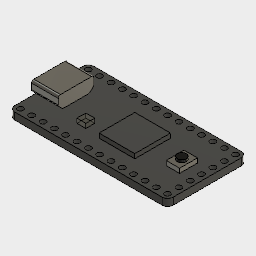
3727 ItsyBitsy M0 (Autodesk Fusion 360 design; units mm, degrees)
Autodesk Fusion 360 part; units mm, degrees
sketch "PCB" plane through (0, 0, 0) normal (0, 0, 1) x (1, 0, 0)
  line L0 (0.508, 6.858) -> (0, 6.35)
  line L1 (0, 16.51) -> (0, 11.684)
  line L2 (0.508, 11.176) -> (0.508, 6.858)
  arc A0 (0, 1.27) -> (1.27, 0) centre (1.27, 1.27) ccw
  line L3 (34.29, 17.78) -> (1.27, 17.78)
  arc A1 (1.27, 17.78) -> (0, 16.51) centre (1.27, 16.51) ccw
  line L4 (35.56, 1.27) -> (35.56, 16.51)
  line L5 (0, 11.684) -> (0.508, 11.176)
  arc A2 (35.56, 16.51) -> (34.29, 17.78) centre (34.29, 16.51) ccw
  line L6 (1.27, 0) -> (34.29, 0)
  arc A3 (34.29, 0) -> (35.56, 1.27) centre (34.29, 1.27) ccw
  line L7 (0, 6.35) -> (0, 1.27)
  circle A4 centre (1.27, 1.27) radius 0.635
  circle A5 centre (1.27, 16.51) radius 0.635
  circle A6 centre (34.29, 3.81) radius 0.635
  circle A7 centre (3.81, 1.27) radius 0.635
  circle A8 centre (3.81, 16.51) radius 0.635
  circle A9 centre (6.35, 1.27) radius 0.635
  circle A10 centre (6.35, 16.51) radius 0.635
  circle A11 centre (8.89, 1.27) radius 0.635
  circle A12 centre (8.89, 16.51) radius 0.635
  circle A13 centre (11.43, 1.27) radius 0.635
  circle A14 centre (11.43, 16.51) radius 0.635
  circle A15 centre (13.97, 1.27) radius 0.635
  circle A16 centre (13.97, 16.51) radius 0.635
  circle A17 centre (16.51, 1.27) radius 0.635
  circle A18 centre (16.51, 16.51) radius 0.635
  circle A19 centre (19.05, 1.27) radius 0.635
  circle A20 centre (19.05, 16.51) radius 0.635
  circle A21 centre (21.59, 1.27) radius 0.635
  circle A22 centre (21.59, 16.51) radius 0.635
  circle A23 centre (24.13, 1.27) radius 0.635
  circle A24 centre (24.13, 16.51) radius 0.635
  circle A25 centre (26.67, 1.27) radius 0.635
  circle A26 centre (26.67, 16.51) radius 0.635
  circle A27 centre (29.21, 1.27) radius 0.635
  circle A28 centre (29.21, 16.51) radius 0.635
  circle A29 centre (31.75, 1.27) radius 0.635
  circle A30 centre (31.75, 16.51) radius 0.635
  circle A31 centre (34.29, 1.27) radius 0.635
  circle A32 centre (34.29, 16.51) radius 0.635
  circle A33 centre (34.29, 6.35) radius 0.635
  circle A34 centre (34.29, 8.89) radius 0.635
  circle A35 centre (34.29, 11.43) radius 0.635
  circle A36 centre (34.29, 13.97) radius 0.635
  dimension "d1" = 1.27
  dimension "d2" = 1.27
  dimension "d3" = 1.27
  dimension "d4" = 1.27
  dimension "d6" = 1.27
  dimension "d7" = 1.27
  dimension "d9" = 1.27
  dimension "d12" = 2.54
  dimension "d13" = 0
  dimension "d16" = 0
  dimension "d17" = 2.54
  measures "d1" diameter of A4
  measures "d2" distance of L6 A0.centre
  measures "d3" distance of L7 A0.centre
  measures "d4" diameter of A5
  measures "d6" distance of L3 A1.centre
  measures "d7" distance of L1 A1.centre
  measures "d9" diameter of A6
extrude "Extrude1" add sketch "PCB" along normal blind 1.6 makes body 1
sketch "microUSB" plane through (0, 0, 1.6) normal (0, 0, 1) x (-1, 0, 0)
  circle A0 centre (-34.29, -1.27) radius 0.635
  circle A1 centre (-34.29, -11.43) radius 0.635
  circle A2 centre (-34.29, -3.81) radius 0.635
  circle A3 centre (-21.59, -16.51) radius 0.635
  circle A4 centre (-3.81, -16.51) radius 0.635
  circle A5 centre (-26.67, -16.51) radius 0.635
  circle A6 centre (-21.59, -1.27) radius 0.635
  circle A7 centre (-6.35, -16.51) radius 0.635
  circle A8 centre (-24.13, -16.51) radius 0.635
  circle A9 centre (-3.81, -1.27) radius 0.635
  circle A10 centre (-16.51, -1.27) radius 0.635
  circle A11 centre (-29.21, -1.27) radius 0.635
  circle A12 centre (-16.51, -16.51) radius 0.635
  circle A13 centre (-1.27, -16.51) radius 0.635
  circle A14 centre (-11.43, -1.27) radius 0.635
  circle A15 centre (-31.75, -16.51) radius 0.635
  circle A16 centre (-11.43, -16.51) radius 0.635
  circle A17 centre (-34.29, -6.35) radius 0.635
  circle A18 centre (-19.05, -1.27) radius 0.635
  circle A19 centre (-8.89, -16.51) radius 0.635
  circle A20 centre (-31.75, -1.27) radius 0.635
  circle A21 centre (-6.35, -1.27) radius 0.635
  circle A22 centre (-29.21, -16.51) radius 0.635
  circle A23 centre (-34.29, -16.51) radius 0.635
  circle A24 centre (-19.05, -16.51) radius 0.635
  circle A25 centre (-13.97, -1.27) radius 0.635
  circle A26 centre (-1.27, -1.27) radius 0.635
  circle A27 centre (-13.97, -16.51) radius 0.635
  circle A28 centre (-8.89, -1.27) radius 0.635
  circle A29 centre (-34.29, -8.89) radius 0.635
  circle A30 centre (-26.67, -1.27) radius 0.635
  circle A31 centre (-34.29, -13.97) radius 0.635
  circle A32 centre (-24.13, -1.27) radius 0.635
  line L0 (0, -6.35) -> (0, -1.27)
  arc A33 (0, -1.27) -> (-1.27, 0) centre (-1.27, -1.27) ccw
  line L1 (-1.27, 0) -> (-34.29, 0)
  arc A34 (-34.29, 0) -> (-35.56, -1.27) centre (-34.29, -1.27) ccw
  line L2 (-35.56, -1.27) -> (-35.56, -16.51)
  arc A35 (-35.56, -16.51) -> (-34.29, -17.78) centre (-34.29, -16.51) ccw
  line L3 (-34.29, -17.78) -> (-1.27, -17.78)
  arc A36 (-1.27, -17.78) -> (0, -16.51) centre (-1.27, -16.51) ccw
  line L4 (0, -16.51) -> (0, -11.684)
  line L5 (0, -11.684) -> (-0.508, -11.176)
  line L6 (-0.508, -11.176) -> (-0.508, -6.858)
  line L7 (-0.508, -6.858) -> (0, -6.35)
  line L8 (0, -13.017) -> (-6, -13.017)
  line L9 (-6, -13.017) -> (-6, -5.017)
  line L10 (-6, -5.017) -> (0, -5.017)
  line L11 (0, -5.017) -> (0, -13.017)
  line L12 (0, -9.017) -> (-6, -9.017) construction
  line L13 (0, -11.684) -> (0, -6.35)
  dimension "d20" = 8
  dimension "d21" = 6
  measures "d20" distance of L8.start L10.end
  measures "d21" distance of L8.start L8.end
extrude "Extrude2" add sketch "microUSB" along normal blind 3 separate body contours L0 L4 L5 L6 L7 L8 L9 L10 L11 | L5 L6 L7 L11 L13 makes body 2
chamfer "Chamfer1" distance 1 angle 45 2 edges at (3, 5.017, 1.6) (3, 13.017, 1.6) on bodies 2
fillet "Fillet1" radius 0.5 6 edges at (3, 5.017, 4.6) (3, 13.017, 4.6) (3, 13.017, 2.6) (3, 12.017, 1.6) (3, 5.017, 2.6) (3, 6.017, 1.6) on bodies 2
shell "Shell1" thickness 0.4 removed faces 1 at (0, 8.086, 3.6) on bodies 2
sketch "SAMD21" plane through (0, 0, 1.6) normal (0, 0, 1) x (-1, 0, 0)
  circle A0 centre (-34.29, -1.27) radius 0.635
  circle A1 centre (-34.29, -11.43) radius 0.635
  circle A2 centre (-34.29, -3.81) radius 0.635
  circle A3 centre (-21.59, -16.51) radius 0.635
  circle A4 centre (-3.81, -16.51) radius 0.635
  circle A5 centre (-26.67, -16.51) radius 0.635
  circle A6 centre (-21.59, -1.27) radius 0.635
  circle A7 centre (-6.35, -16.51) radius 0.635
  circle A8 centre (-24.13, -16.51) radius 0.635
  circle A9 centre (-3.81, -1.27) radius 0.635
  circle A10 centre (-16.51, -1.27) radius 0.635
  circle A11 centre (-29.21, -1.27) radius 0.635
  circle A12 centre (-16.51, -16.51) radius 0.635
  circle A13 centre (-1.27, -16.51) radius 0.635
  circle A14 centre (-11.43, -1.27) radius 0.635
  circle A15 centre (-31.75, -16.51) radius 0.635
  circle A16 centre (-11.43, -16.51) radius 0.635
  circle A17 centre (-34.29, -6.35) radius 0.635
  circle A18 centre (-19.05, -1.27) radius 0.635
  circle A19 centre (-8.89, -16.51) radius 0.635
  circle A20 centre (-31.75, -1.27) radius 0.635
  circle A21 centre (-6.35, -1.27) radius 0.635
  circle A22 centre (-29.21, -16.51) radius 0.635
  circle A23 centre (-34.29, -16.51) radius 0.635
  circle A24 centre (-19.05, -16.51) radius 0.635
  circle A25 centre (-13.97, -1.27) radius 0.635
  circle A26 centre (-1.27, -1.27) radius 0.635
  circle A27 centre (-13.97, -16.51) radius 0.635
  circle A28 centre (-8.89, -1.27) radius 0.635
  circle A29 centre (-34.29, -8.89) radius 0.635
  circle A30 centre (-26.67, -1.27) radius 0.635
  circle A31 centre (-34.29, -13.97) radius 0.635
  circle A32 centre (-24.13, -1.27) radius 0.635
  line L0 (0, -6.35) -> (0, -1.27)
  arc A33 (0, -1.27) -> (-1.27, 0) centre (-1.27, -1.27) ccw
  line L1 (-1.27, 0) -> (-34.29, 0)
  arc A34 (-34.29, 0) -> (-35.56, -1.27) centre (-34.29, -1.27) ccw
  line L2 (-35.56, -1.27) -> (-35.56, -16.51)
  arc A35 (-35.56, -16.51) -> (-34.29, -17.78) centre (-34.29, -16.51) ccw
  line L3 (-34.29, -17.78) -> (-1.27, -17.78)
  arc A36 (-1.27, -17.78) -> (0, -16.51) centre (-1.27, -16.51) ccw
  line L4 (0, -16.51) -> (0, -11.684)
  line L5 (0, -11.684) -> (-0.508, -11.176)
  line L6 (-0.508, -11.176) -> (-0.508, -6.858)
  line L7 (-0.508, -6.858) -> (0, -6.35)
  line L8 (-23.812, -4.382) -> (-15.812, -4.382)
  line L9 (-15.812, -4.382) -> (-15.812, -12.382)
  line L10 (-15.812, -12.382) -> (-23.812, -12.382)
  line L11 (-23.812, -12.382) -> (-23.812, -4.382)
  line L12 (-23.812, -4.382) -> (-15.812, -12.382) construction
  line L13 (-15.812, -4.382) -> (-23.812, -12.382) construction
  point P0 (-19.812, -8.382)
  dimension "d28" = 8
  dimension "d29" = 8
  dimension "d30" = 19.812
  dimension "d31" = 8.382
  measures "d28" distance of L9.end L10.end
  measures "d29" distance of L8.end L9.end
  measures "d30" distance of L0 P0
  measures "d31" distance of L1 P0
extrude "Extrude3" add sketch "SAMD21" along normal blind 1 separate body contours L8 L9 L10 L11 makes body 3
sketch "reset" plane through (0, 0, 1.6) normal (0, 0, 1) x (-1, 0, 0)
  circle A0 centre (-34.29, -1.27) radius 0.635
  circle A1 centre (-34.29, -11.43) radius 0.635
  circle A2 centre (-34.29, -3.81) radius 0.635
  circle A3 centre (-21.59, -16.51) radius 0.635
  circle A4 centre (-3.81, -16.51) radius 0.635
  circle A5 centre (-26.67, -16.51) radius 0.635
  circle A6 centre (-21.59, -1.27) radius 0.635
  circle A7 centre (-6.35, -16.51) radius 0.635
  circle A8 centre (-24.13, -16.51) radius 0.635
  circle A9 centre (-3.81, -1.27) radius 0.635
  circle A10 centre (-16.51, -1.27) radius 0.635
  circle A11 centre (-29.21, -1.27) radius 0.635
  circle A12 centre (-16.51, -16.51) radius 0.635
  circle A13 centre (-1.27, -16.51) radius 0.635
  circle A14 centre (-11.43, -1.27) radius 0.635
  circle A15 centre (-31.75, -16.51) radius 0.635
  circle A16 centre (-11.43, -16.51) radius 0.635
  circle A17 centre (-34.29, -6.35) radius 0.635
  circle A18 centre (-19.05, -1.27) radius 0.635
  circle A19 centre (-8.89, -16.51) radius 0.635
  circle A20 centre (-31.75, -1.27) radius 0.635
  circle A21 centre (-6.35, -1.27) radius 0.635
  circle A22 centre (-29.21, -16.51) radius 0.635
  circle A23 centre (-34.29, -16.51) radius 0.635
  circle A24 centre (-19.05, -16.51) radius 0.635
  circle A25 centre (-13.97, -1.27) radius 0.635
  circle A26 centre (-1.27, -1.27) radius 0.635
  circle A27 centre (-13.97, -16.51) radius 0.635
  circle A28 centre (-8.89, -1.27) radius 0.635
  circle A29 centre (-34.29, -8.89) radius 0.635
  circle A30 centre (-26.67, -1.27) radius 0.635
  circle A31 centre (-34.29, -13.97) radius 0.635
  circle A32 centre (-24.13, -1.27) radius 0.635
  line L0 (0, -6.35) -> (0, -1.27)
  arc A33 (0, -1.27) -> (-1.27, 0) centre (-1.27, -1.27) ccw
  line L1 (-1.27, 0) -> (-34.29, 0)
  arc A34 (-34.29, 0) -> (-35.56, -1.27) centre (-34.29, -1.27) ccw
  line L2 (-35.56, -1.27) -> (-35.56, -16.51)
  arc A35 (-35.56, -16.51) -> (-34.29, -17.78) centre (-34.29, -16.51) ccw
  line L3 (-34.29, -17.78) -> (-1.27, -17.78)
  arc A36 (-1.27, -17.78) -> (0, -16.51) centre (-1.27, -16.51) ccw
  line L4 (0, -16.51) -> (0, -11.684)
  line L5 (0, -11.684) -> (-0.508, -11.176)
  line L6 (-0.508, -11.176) -> (-0.508, -6.858)
  line L7 (-0.508, -6.858) -> (0, -6.35)
  line L8 (-31.6625, -6.5725) -> (-28.6625, -6.5725)
  line L9 (-28.6625, -6.5725) -> (-28.6625, -10.5725)
  line L10 (-28.6625, -10.5725) -> (-31.6625, -10.5725)
  line L11 (-31.6625, -10.5725) -> (-31.6625, -6.5725)
  line L12 (-31.6625, -6.5725) -> (-28.6625, -10.5725) construction
  line L13 (-28.6625, -6.5725) -> (-31.6625, -10.5725) construction
  circle A37 centre (-30.1625, -8.5725) radius 1
  point P0 (-30.1625, -8.5725)
  dimension "d34" = 3
  dimension "d35" = 4
  dimension "d36" = 2
  dimension "d37" = 30.1625
  dimension "d38" = 8.5725
  measures "d34" distance of L9.end L10.end
  measures "d35" distance of L8.end L9.end
  measures "d36" diameter of A37
  measures "d37" distance of L0 P0
  measures "d38" distance of L1 P0
extrude "Extrude4" add sketch "reset" along normal blind 1 separate body contours L8 L9 L10 L11 | A37 makes body 4
extrude "Extrude5" add sketch "reset" along normal blind 0.6 from surface at 1 contours A37 bodies 4
sketch "DotStar APA102" plane through (0, 0, 1.6) normal (0, 0, 1) x (-1, 0, 0)
  circle A0 centre (-34.29, -1.27) radius 0.635
  circle A1 centre (-34.29, -11.43) radius 0.635
  circle A2 centre (-34.29, -3.81) radius 0.635
  circle A3 centre (-21.59, -16.51) radius 0.635
  circle A4 centre (-3.81, -16.51) radius 0.635
  circle A5 centre (-26.67, -16.51) radius 0.635
  circle A6 centre (-21.59, -1.27) radius 0.635
  circle A7 centre (-6.35, -16.51) radius 0.635
  circle A8 centre (-24.13, -16.51) radius 0.635
  circle A9 centre (-3.81, -1.27) radius 0.635
  circle A10 centre (-16.51, -1.27) radius 0.635
  circle A11 centre (-29.21, -1.27) radius 0.635
  circle A12 centre (-16.51, -16.51) radius 0.635
  circle A13 centre (-1.27, -16.51) radius 0.635
  circle A14 centre (-11.43, -1.27) radius 0.635
  circle A15 centre (-31.75, -16.51) radius 0.635
  circle A16 centre (-11.43, -16.51) radius 0.635
  circle A17 centre (-34.29, -6.35) radius 0.635
  circle A18 centre (-19.05, -1.27) radius 0.635
  circle A19 centre (-8.89, -16.51) radius 0.635
  circle A20 centre (-31.75, -1.27) radius 0.635
  circle A21 centre (-6.35, -1.27) radius 0.635
  circle A22 centre (-29.21, -16.51) radius 0.635
  circle A23 centre (-34.29, -16.51) radius 0.635
  circle A24 centre (-19.05, -16.51) radius 0.635
  circle A25 centre (-13.97, -1.27) radius 0.635
  circle A26 centre (-1.27, -1.27) radius 0.635
  circle A27 centre (-13.97, -16.51) radius 0.635
  circle A28 centre (-8.89, -1.27) radius 0.635
  circle A29 centre (-34.29, -8.89) radius 0.635
  circle A30 centre (-26.67, -1.27) radius 0.635
  circle A31 centre (-34.29, -13.97) radius 0.635
  circle A32 centre (-24.13, -1.27) radius 0.635
  line L0 (0, -6.35) -> (0, -1.27)
  arc A33 (0, -1.27) -> (-1.27, 0) centre (-1.27, -1.27) ccw
  line L1 (-1.27, 0) -> (-34.29, 0)
  arc A34 (-34.29, 0) -> (-35.56, -1.27) centre (-34.29, -1.27) ccw
  line L2 (-35.56, -1.27) -> (-35.56, -16.51)
  arc A35 (-35.56, -16.51) -> (-34.29, -17.78) centre (-34.29, -16.51) ccw
  line L3 (-34.29, -17.78) -> (-1.27, -17.78)
  arc A36 (-1.27, -17.78) -> (0, -16.51) centre (-1.27, -16.51) ccw
  line L4 (0, -16.51) -> (0, -11.684)
  line L5 (0, -11.684) -> (-0.508, -11.176)
  line L6 (-0.508, -11.176) -> (-0.508, -6.858)
  line L7 (-0.508, -6.858) -> (0, -6.35)
  line L8 (-12.43, -4.7785) -> (-10.43, -4.7785)
  line L9 (-10.43, -4.7785) -> (-10.43, -6.7785)
  line L10 (-10.43, -6.7785) -> (-12.43, -6.7785)
  line L11 (-12.43, -6.7785) -> (-12.43, -4.7785)
  line L12 (-12.43, -4.7785) -> (-10.43, -6.7785) construction
  line L13 (-10.43, -4.7785) -> (-12.43, -6.7785) construction
  point P0 (-11.43, -5.7785)
  dimension "d44" = 2
  dimension "d45" = 2
  dimension "d46" = 11.43
  dimension "d47" = 5.7785
  measures "d44" distance of L8.end L9.end
  measures "d45" distance of L9.end L10.end
  measures "d46" distance of L0 P0
  measures "d47" distance of L1 P0
extrude "Extrude6" add sketch "DotStar APA102" along normal blind 1 separate body contours L8 L9 L10 L11 makes body 5
equation "d1 = pins"
equation "d4 = pins"
equation "pins = 1.27 mm"
equation "d9 = pins"
equation "d12 = pins * 2"
equation "d17 = pins * 2"
named bodies: "PCB", "USB", "samd21", "reset", "DotStar"
